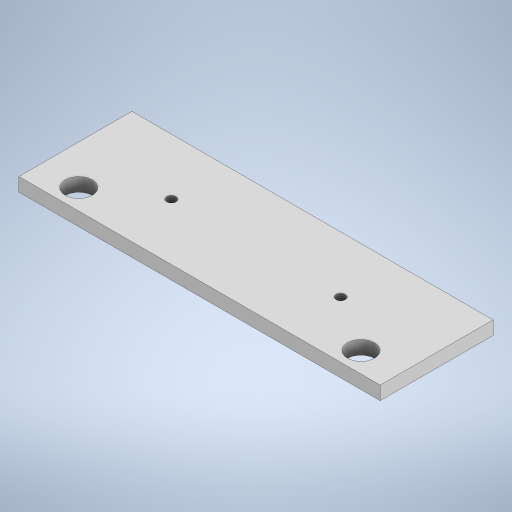
# Autodesk Inventor part: Joining Brace Front
Saved by Autodesk Inventor 2023.2 (Build 272271000, 271)
## iProperties
Created: 2023-02-15
Part Number: Joining Brace Front
Material: Generic
Document SubType Name: Modeling
Designer: dmargari
Density: 1 g/cm^3
Appearance: Default
Author: dmargari
Autodesk Inventor part; units mm, degrees
ref_plane "YZ Plane" through (0, 0, 0) normal (1, 0, 0) x (0, 1, 0)
ref_plane "XZ Plane" through (0, 0, 0) normal (0, 1, 0) x (-1, 0, 0)
ref_plane "XY Plane" through (0, 0, 0) normal (0, 0, 1) x (1, 0, 0)
sketch "Sketch1" plane through (0, 0, 0) normal (0, 1, 0) x (-1, 0, 0)
  line L0 (25.2233, -4.8143) -> (-134.7767, -4.8143)
  line L1 (-134.7767, -4.8143) -> (-134.7767, -54.8143)
  line L2 (-134.7767, -54.8143) -> (25.2233, -54.8143)
  line L3 (25.2233, -54.8143) -> (25.2233, -4.8143)
  line L4 (25.2233, -13.8143) -> (-134.7767, -13.8143) construction
  circle A0 centre (7.7233, -13.8143) radius 6
  circle A1 centre (-117.2767, -13.8143) radius 6
  point P0 (0, 0)
  dimension "d0" = 160
  dimension "d1" = 50
  dimension "d2" = 9
  dimension "d3" = 12
  dimension "d4" = 12
  dimension "d5" = 125
  dimension "d6" = 17.5
  constraints: 10 end point, 4 point on line, 2 centre point, 2 parallel, 2 perpendicular, 1 horizontal
  measures "d0" distance of L2.end L1.end
  measures "d1" distance of L1.end L0.end
  measures "d2" distance between parallel lines of L4 L0
  measures "d3" diameter of A0
  measures "d4" diameter of A1
  measures "d5" distance of A0.centre A1.centre
  measures "d6" distance from line of L3 A0.centre
extrude "Extrusion1" add sketch "Sketch1" along normal blind 6
sketch "Sketch2" plane through (0, 6, 0) normal (0, 1, 0) x (1, 0, 0)
  line L0 (-25.2233, 54.8143) -> (-25.2233, 4.8143) construction
  line L1 (-25.2233, 29.8143) -> (134.7767, 29.8143) construction
  line L2 (134.7767, 4.8143) -> (134.7767, 54.8143) construction
  circle A0 centre (17.2767, 29.8143) radius 2.4
  circle A1 centre (92.2767, 29.8143) radius 2.4
  point P0 (0, 0)
  dimension "d9" = 4.8
  dimension "d10" = 4.8
  dimension "d11" = 75
  dimension "d12" = 42.5
  constraints: 2 centre point, 2 end point, 2 midpoint, 2 point on line
  measures "d9" diameter of A0
  measures "d10" diameter of A1
  measures "d11" distance of A1.centre A0.centre
  measures "d12" distance from line of A0.centre L0
hole "Hole1" at (92.2767, 6, -29.8143) at (17.2767, 6, -29.8143) direction (0, -1, 0) diameter 4.134 depth 6 tip angle 118 thread size "M5x0.8" class "6H" standard "ISO Metric profile"
body "Solid1"
